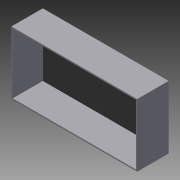
# Autodesk Inventor part: electrical shelfing
Saved by Autodesk Inventor 2012 SP1 (Build 160190100, 190)
## iProperties
Created: 2012-01-27
Part Number: electrical shelfing
Material: Aluminum-6061
Document SubType Name: Modeling
Designer: adamides odysseus
Density: 2.71 g/cm^3
Mass: 7729.93 g
Surface Area: 9099.98 cm^2
Volume: 2852.37 cm^3
Author: adamides odysseus
Autodesk Inventor part; units mm, degrees
ref_plane "YZ Plane" through (0, 0, 0) normal (1, 0, 0) x (0, 1, 0)
ref_plane "XZ Plane" through (0, 0, 0) normal (0, 1, 0) x (-1, 0, 0)
ref_plane "XY Plane" through (0, 0, 0) normal (0, 0, 1) x (1, 0, 0)
sketch "Sketch1" plane through (0, 0, 0) normal (0, 0, 1) x (1, 0, 0)
  line L0 (0, 0) -> (609.6, 0)
  line L1 (609.6, 0) -> (609.6, 304.8)
  line L2 (609.6, 304.8) -> (0, 304.8)
  line L3 (0, 304.8) -> (0, 0)
  dimension "d0" = 609.6
  dimension "d1" = 304.8
  constraints: 8 end point, 2 parallel, 1 horizontal, 1 perpendicular
  measures "d0" distance of L1.end L2.end
  measures "d1" distance of L0.end L1.end
extrude "Extrusion1" add sketch "Sketch1" along normal blind 152.4
sketch "Sketch2" plane through (0, 0, 152.4) normal (0, 0, 1) x (1, 0, 0)
  line L0 (0, 0) -> (0, 304.8) projected
  line L1 (609.6, 0) -> (0, 0) projected
  line L2 (609.6, 304.8) -> (609.6, 0) projected
  line L3 (0, 304.8) -> (609.6, 304.8) projected
  line L4 (6.35, 6.35) -> (603.25, 6.35)
  line L5 (603.25, 6.35) -> (603.25, 298.45)
  line L6 (603.25, 298.45) -> (6.35, 298.45)
  line L7 (6.35, 298.45) -> (6.35, 6.35)
  dimension "d4" = 6.35
  dimension "d5" = 6.35
  dimension "d6" = 6.35
  dimension "d7" = 6.35
  constraints: 8 end point, 2 parallel, 1 horizontal, 1 perpendicular
  measures "d4" distance between parallel lines of L3 L6
  measures "d5" distance between parallel lines of L0 L7
  measures "d6" distance between parallel lines of L2 L5
  measures "d7" distance between parallel lines of L1 L4
extrude "Extrusion2" cut sketch "Sketch2" against normal blind 146.05 contours L7 L6 L5 L4
body "Solid1"
